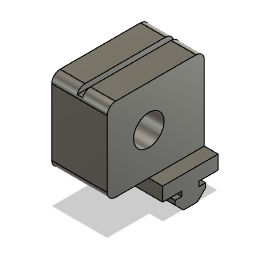
wire+mover (Autodesk Fusion 360 design; units mm, degrees)
Autodesk Fusion 360 part; units mm, degrees
sketch "Sketch1" plane through (0, 0, 0) normal (1, 0, 0) x (0, 0, -1)
  line L0 (0, 0) -> (2.5225, 0)
  line L1 (2.5225, 0) -> (5.5, 2.98)
  line L2 (5.5, 2.98) -> (5.5, 4.5)
  line L3 (5.5, 4.5) -> (3.1, 4.5)
  line L4 (3.1, 4.5) -> (3.1, 6.2)
  line L5 (3.1, 6.2) -> (10, 6.2)
  line L6 (10, 6.2) -> (10, 11.2)
  line L7 (10, 11.2) -> (0, 11.2)
  line L8 (0, 0) -> (0, 21.3117) construction
  line L9 (-10, 6.2) -> (-10, 11.2)
  line L10 (0, 0) -> (-2.5225, 0)
  line L11 (-3.1, 6.2) -> (-10, 6.2)
  line L12 (-5.5, 2.98) -> (-5.5, 4.5)
  line L13 (-10, 11.2) -> (0, 11.2)
  line L14 (-5.5, 4.5) -> (-3.1, 4.5)
  line L15 (-2.5225, 0) -> (-5.5, 2.98)
  line L16 (-3.1, 4.5) -> (-3.1, 6.2)
  dimension "d3" = 2.5225
  dimension "d4" = 4.5
  dimension "d6" = 2.4
  dimension "d7" = 3.1
  dimension "d8" = 1.52
  dimension "d9" = 1.7
  dimension "d10" = 5
  dimension "d11" = 10
  constraint coincident L0.start L8.start
  constraint horizontal L0
  constraint perpendicular L0 L2
  constraint perpendicular L2 L3
  constraint perpendicular L0 L4
  constraint perpendicular L4 L5
  constraint perpendicular L5 L6
  constraint perpendicular L6 L7
  constraint perpendicular L7 L8
  constraint symmetric L0.start L8 L10.start
  constraint symmetric L0.end L8 L10.end
  constraint symmetric L1.end L8 L12.start
  constraint symmetric L2.end L8 L12.end
  constraint symmetric L3.end L8 L14.end
  constraint symmetric L4.end L8 L11.start
  constraint symmetric L5.end L8 L9.start
  constraint symmetric L6.end L8 L9.end
  constraint symmetric L7.end L8 L13.end
  constraint coincident L7.end L8
  measures "d3" distance of L0.start L0.end
  measures "d4" distance of L0 L3
  measures "d6" distance of L2.end L3.end
  measures "d7" distance of L4 L8
  measures "d8" distance of L1.end L2.end
  measures "d9" distance of L3.end L4.end
  measures "d10" distance of L5.end L6.end
  measures "d11" distance of L6.end L7.end
extrude "Extrude1" add sketch "Sketch1" along normal blind 30
ref_plane "WorkPlane1" through (15, 5.6, 0) normal (1, 0, 0) x (0, 0, -1)
sketch "Sketch2" plane through (15, 5.6, 0) normal (1, 0, 0) x (0, 0, -1)
  line L0 (10, 5.6) -> (-10, 5.6)
  line L1 (10, 5.6) -> (-22, 5.6)
  line L2 (-25, 8.6) -> (-25, 32.6)
  line L3 (-22, 35.6) -> (7, 35.6)
  line L4 (10, 32.6) -> (10, 5.6)
  circle A0 centre (-10, 20.6) radius 11.5
  line L5 (-25, 20.6) -> (10, 20.6) construction
  circle A1 centre (-10, 20.6) radius 5.5
  arc A2 (-22, 35.6) -> (-25, 32.6) centre (-22, 32.6) ccw
  arc A3 (10, 32.6) -> (7, 35.6) centre (7, 32.6) ccw
  arc A4 (-25, 8.6) -> (-22, 5.6) centre (-22, 8.6) ccw
  point P0 (-25, 5.6)
  point P1 (10, 35.6)
  dimension "d15" = 35
  dimension "d16" = 30
  dimension "d17" = 23
  dimension "d18" = 15
  dimension "d19" = 11
  dimension "d29" = 3
  dimension "d30" = 3
  constraint horizontal L1
  constraint vertical L2
  constraint horizontal L3
  constraint vertical L4
  constraint coincident L0.start L1.start
  constraint coincident A0.centre L5
  constraint concentric A0 A1
  constraint coincident L2 L5.start
  constraint tangent L2 A2
  constraint tangent L3 A2
  constraint coincident L4 L5.end
  constraint coincident P1 L3
  constraint coincident P1 L4
  constraint tangent L3 A3
  constraint tangent L4 A3
  constraint equal A2 A3
  constraint coincident P0 L2
  constraint coincident P0 L1
  constraint tangent L2 A4
  constraint tangent L1 A4
  measures "d15" distance of L0.start P0
  measures "d16" distance of L0.start P1
  measures "d17" diameter of A0
  measures "d18" distance of L2 A0.centre
  measures "d19" diameter of A1
  measures "d29" radius of A4
  measures "d30" radius of A2
extrude "Extrude2" add sketch "Sketch2" along normal blind 10 and the other way blind 10 contours L0 L1 L2 L3 L4 A2 A3 A4
extrude "Extrude3" add sketch "Sketch2" along normal blind 10 and the other way blind 6 contours A0
sketch "Sketch3" plane through (0, 0, 25) normal (0, 0, 1) x (1, 0, 0)
  line L0 (5, 14.2) -> (25, 14.2)
  line L1 (25, 14.2) -> (25, 38.2)
  line L2 (25, 38.2) -> (5, 38.2)
  line L3 (5, 38.2) -> (5, 14.2)
  line L4 (25, 41.2) -> (5, 41.2)
  line L5 (14, 41.2) -> (16, 41.2)
  line L6 (16, 41.2) -> (16, 39.2)
  line L7 (16, 39.2) -> (14, 39.2)
  line L8 (14, 39.2) -> (14, 41.2)
  dimension "d31" = 2
  dimension "d32" = 2
  constraint horizontal L5
  constraint vertical L6
  constraint horizontal L7
  constraint vertical L8
  constraint coincident L4 L5.start
  measures "d31" distance of L5.start L5.end
  measures "d32" distance of L5.start L7.end
extrude "Extrude4" cut sketch "Sketch3" against normal through all contours L4 L5 L6 L7 L8
